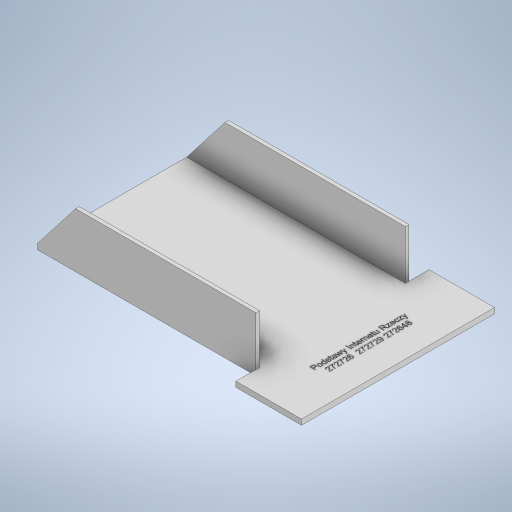
# Autodesk Inventor part: Część1
Saved by Autodesk Inventor 2024 (Build 280153020, 153B)
## iProperties
Created: 2025-01-23
Part Number: Część1
Material: Ogólny
Document SubType Name: Modeling
Designer: jakub
Density: 1 g/cm^3
Appearance: Domyślna
Author: jakub
Autodesk Inventor part; units mm, degrees
(part 1 of 2)
ref_plane "YZ Plane" through (0, 0, 0) normal (1, 0, 0) x (0, 1, 0)
ref_plane "XZ Plane" through (0, 0, 0) normal (0, 1, 0) x (-1, 0, 0)
ref_plane "XY Plane" through (0, 0, 0) normal (0, 0, 1) x (1, 0, 0)
sketch "Szkic1" plane through (0, 0, 0) normal (0, 1, 0) x (-1, 0, 0)
  line L0 (-24, 40) -> (60, 40)
  line L1 (60, -40) -> (-24, -40)
  line L2 (-60, -40) -> (-60, 40)
  line L3 (-60, 40) -> (60, -40) construction
  line L4 (60, 40) -> (-60, -40) construction
  line L5 (-24, -40) -> (-24, -53)
  line L6 (-24, -53) -> (-60, -53)
  line L7 (-60, -53) -> (-60, -40)
  line L8 (-24, 40) -> (-24, 53)
  line L9 (-24, 53) -> (-60, 53)
  line L10 (-60, 53) -> (-60, 40)
  line L11 (60, -40) -> (96, -40)
  line L12 (96, -40) -> (96, 40)
  line L13 (96, 40) -> (60, 40)
  point P0 (0, 0)
  dimension "d0" = 120
  dimension "d1" = 80
  dimension "d6" = 106
  dimension "d7" = 84
  dimension "d8" = 84
  dimension "d9" = 13
  dimension "d10" = 13
  dimension "d11" = 40
  dimension "d12" = 53
  dimension "d16" = 36
  dimension "d17" = 80
  dimension "d18" = 156
  constraints: 28 end point, 4 parallel, 2 horizontal, 2 midpoint, 1 perpendicular
  measures "d0" distance of L1.start L2.start
  measures "d1" distance of L0.end L1.start
  measures "d6" distance between parallel lines of L6 L9
  measures "d7" distance of L0.start L0.end
  measures "d8" distance of L1.start L1.end
  measures "d9" distance of L0.start L8.end
  measures "d10" distance of L1.end L5.end
  measures "d11" distance from line of point (0, 0) L1
  measures "d12" distance from line of point (0, 0) L9
  measures "d16" distance of L13.end L12.end
  measures "d17" distance of L11.end L12.end
  measures "d18" distance between parallel lines of L2 L12
extrude "Wyciągnięcie proste1" add sketch "Szkic1" along normal blind 3
sketch "Szkic2" plane through (0, 0, 0) normal (0, -1, 0) x (1, 0, 0)
  line L0 (24, -40) -> (-96, -40)
  line L1 (-96, -40) -> (-96, -42)
  line L2 (-96, -42) -> (24, -42)
  line L3 (24, -42) -> (24, -40)
  line L4 (24, 40) -> (-96, 40)
  line L5 (-96, 40) -> (-96, 42)
  line L6 (-96, 42) -> (24, 42)
  line L7 (24, 42) -> (24, 40)
  point P0 (0, 0)
  dimension "d19" = 2
  dimension "d20" = 120
  dimension "d21" = 2
  constraints: 16 end point, 4 parallel, 2 horizontal, 2 perpendicular, 1 point on line
  measures "d19" distance of L1.end L0.end
  measures "d20" distance of L5.end L6.end
  measures "d21" distance of L4.end L5.end
extrude "Wyciągnięcie proste2" add sketch "Szkic2" against normal blind 30
sketch "Szkic7" plane through (-96, 3, -40) normal (0, 0, 1) x (1, 0, 0)
  line L0 (0, 27) -> (120, 27) projected
  line L1 (0, 0) -> (21, 27)
  line L2 (0, 27) -> (21, 27)
  line L3 (0, 0) -> (0, 27)
  point P0 (96, -3)
  constraints: 6 end point, 1 perpendicular, 1 point on line
extrude "Wyciągnięcie proste4" cut sketch "Szkic7" along normal mid plane 200
sketch "Szkic8" plane through (0, 3, 0) normal (0, 1, 0) x (1, 0, 0)
  line L0 (37.3604, -27.9644) -> (37.3604, 27.055) construction
  line L1 (37.3604, 27.055) -> (143.5342, 27.055) construction
  line L2 (143.5342, 27.055) -> (143.5342, -27.9644) construction
  line L3 (143.5342, -27.9644) -> (37.3604, -27.9644) construction
  line L4 (40.4104, -25.9403) -> (37.3604, -25.9403)
  line L5 (37.3604, -25.9403) -> (37.3604, -24.7896)
  spline S0 degree 2 poles (37.3604, -24.7896) (37.3604, -24.4851) (37.3907, -24.3247) knots 0 0 0 1 1 1
  spline S1 degree 2 poles (37.3907, -24.3247) (37.4278, -24.0992) (37.6371, -23.797) (38.016, -23.611) (38.2438, -23.611) knots 0 0 0 1 2 3 3 3
  spline S2 degree 2 poles (38.2438, -23.611) (38.632, -23.611) (39.1714, -24.1062) (39.1714, -24.7524) knots 0 0 0 1 2 2 2
  line L6 (39.1714, -24.7524) -> (39.1714, -25.5358)
  line L7 (39.1714, -25.5358) -> (40.4104, -25.5358)
  line L8 (40.4104, -25.5358) -> (40.4104, -25.9403)
  line L9 (38.811, -25.5358) -> (38.811, -24.7478)
  spline S3 degree 2 poles (38.811, -24.7478) (38.811, -24.3549) (38.5205, -24.0271) (38.2554, -24.0271) knots 0 0 0 1 2 2 2
  spline S4 degree 2 poles (38.2554, -24.0271) (38.0648, -24.0271) (37.7905, -24.2201) (37.7487, -24.3781) knots 0 0 0 1 2 2 2
  spline S5 degree 2 poles (37.7487, -24.3781) (37.7208, -24.4804) (37.7208, -24.7547) knots 0 0 0 1 1 1
  line L10 (37.7208, -24.7547) -> (37.7208, -25.5358)
  line L11 (37.7208, -25.5358) -> (38.811, -25.5358)
  spline S6 degree 2 poles (39.3039, -23.2832) (38.6925, -23.2832) (38.3972, -22.9415) knots 0 0 0 1 1 1
  spline S7 degree 2 poles (38.3972, -22.9415) (38.1508, -22.6579) (38.1508, -22.2487) knots 0 0 0 1 1 1
  spline S8 degree 2 poles (38.1508, -22.2487) (38.1508, -21.7931) (38.7483, -21.2142) (39.2737, -21.2142) knots 0 0 0 1 2 2 2
  spline S9 degree 2 poles (39.2737, -21.2142) (39.6991, -21.2142) (40.1896, -21.47) (40.4592, -21.9581) (40.4592, -22.2487) knots 0 0 0 1 2 3 3 3
  spline S10 degree 2 poles (40.4592, -22.2487) (40.4592, -22.7113) (39.8641, -23.2832) (39.3039, -23.2832) knots 0 0 0 1 2 2 2
  spline S11 degree 2 poles (39.3062, -22.8973) (39.7293, -22.8973) (40.1524, -22.5277) (40.1524, -22.2487) knots 0 0 0 1 2 2 2
  spline S12 degree 2 poles (40.1524, -22.2487) (40.1524, -21.9698) (39.727, -21.6001) (39.2923, -21.6001) knots 0 0 0 1 2 2 2
  spline S13 degree 2 poles (39.2923, -21.6001) (38.8831, -21.6001) (38.46, -21.9721) (38.46, -22.2487) knots 0 0 0 1 2 2 2
  spline S14 degree 2 poles (38.46, -22.2487) (38.46, -22.5277) (38.8808, -22.8973) (39.3062, -22.8973) knots 0 0 0 1 2 2 2
  line L12 (40.4104, -19.3405) -> (40.1315, -19.3405)
  spline S15 degree 2 poles (40.1315, -19.3405) (40.4592, -19.5498) (40.4592, -19.9589) knots 0 0 0 1 1 1
  spline S16 degree 2 poles (40.4592, -19.9589) (40.4592, -20.2239) (40.1687, -20.6656) (39.6456, -20.9097) (39.3062, -20.9097) knots 0 0 0 1 2 3 3 3
  spline S17 degree 2 poles (39.3062, -20.9097) (38.9761, -20.9097) (38.4368, -20.6889) (38.1508, -20.2495) (38.1508, -19.9775) knots 0 0 0 1 2 3 3 3
  spline S18 degree 2 poles (38.1508, -19.9775) (38.1508, -19.7776) (38.3182, -19.4661) (38.453, -19.3684) knots 0 0 0 1 2 2 2
  line L13 (38.453, -19.3684) -> (37.3604, -19.3684)
  line L14 (37.3604, -19.3684) -> (37.3604, -18.9941)
  line L15 (37.3604, -18.9941) -> (40.4104, -18.9941)
  line L16 (40.4104, -18.9941) -> (40.4104, -19.3405)
  spline S19 degree 2 poles (39.3062, -20.5238) (39.7316, -20.5238) (40.1524, -20.1658) (40.1524, -19.9217) knots 0 0 0 1 2 2 2
  spline S20 degree 2 poles (40.1524, -19.9217) (40.1524, -19.6776) (39.7502, -19.3336) (39.3387, -19.3336) knots 0 0 0 1 2 2 2
  spline S21 degree 2 poles (39.3387, -19.3336) (38.8854, -19.3336) (38.46, -19.6823) (38.46, -19.938) knots 0 0 0 1 2 2 2
  spline S22 degree 2 poles (38.46, -19.938) (38.46, -20.189) (38.8692, -20.5238) (39.3062, -20.5238) knots 0 0 0 1 2 2 2
  line L17 (39.7502, -18.5571) -> (39.6921, -18.1875)
  spline S23 degree 2 poles (39.6921, -18.1875) (39.9153, -18.1573) (40.1524, -17.8713) (40.1524, -17.6133) knots 0 0 0 1 2 2 2
  spline S24 degree 2 poles (40.1524, -17.6133) (40.1524, -17.3552) (39.9408, -17.1042) (39.799, -17.1042) knots 0 0 0 1 2 2 2
  spline S25 degree 2 poles (39.799, -17.1042) (39.6735, -17.1042) (39.5991, -17.2158) knots 0 0 0 1 1 1
  spline S26 degree 2 poles (39.5991, -17.2158) (39.5503, -17.2925) (39.4736, -17.5993) knots 0 0 0 1 1 1
  spline S27 degree 2 poles (39.4736, -17.5993) (39.369, -18.0108) (39.2179, -18.3293) (38.9482, -18.4943) (38.7878, -18.4943) knots 0 0 0 1 2 3 3 3
  spline S28 degree 2 poles (38.7878, -18.4943) (38.639, -18.4943) (38.3879, -18.3595) (38.3043, -18.2433) knots 0 0 0 1 2 2 2
  spline S29 degree 2 poles (38.3043, -18.2433) (38.2392, -18.1549) (38.1508, -17.8527) (38.1508, -17.6784) knots 0 0 0 1 2 2 2
  spline S30 degree 2 poles (38.1508, -17.6784) (38.1508, -17.418) (38.3019, -17.0251) (38.5576, -16.8368) (38.7715, -16.802) knots 0 0 0 1 2 3 3 3
  line L18 (38.7715, -16.802) -> (38.8203, -17.1693)
  spline S31 degree 2 poles (38.8203, -17.1693) (38.6483, -17.1948) (38.4577, -17.4343) (38.4577, -17.6528) knots 0 0 0 1 2 2 2
  spline S32 degree 2 poles (38.4577, -17.6528) (38.4577, -17.9108) (38.6297, -18.1317) (38.7436, -18.1317) knots 0 0 0 1 2 2 2
  spline S33 degree 2 poles (38.7436, -18.1317) (38.8157, -18.1317) (38.8738, -18.0852) knots 0 0 0 1 1 1
  spline S34 degree 2 poles (38.8738, -18.0852) (38.9342, -18.041) (38.9738, -17.9411) knots 0 0 0 1 1 1
  spline S35 degree 2 poles (38.9738, -17.9411) (38.9947, -17.8853) (39.0714, -17.611) knots 0 0 0 1 1 1
  spline S36 degree 2 poles (39.0714, -17.611) (39.176, -17.2134) (39.3109, -16.8973) (39.5689, -16.7183) (39.7618, -16.7183) knots 0 0 0 1 2 3 3 3
  spline S37 degree 2 poles (39.7618, -16.7183) (39.9478, -16.7183) (40.2779, -16.9368) (40.4592, -17.3506) (40.4592, -17.611) knots 0 0 0 1 2 3 3 3
  spline S38 degree 2 poles (40.4592, -17.611) (40.4592, -18.041) (40.1012, -18.4943) (39.7502, -18.5571) knots 0 0 0 1 2 2 2
  line L19 (40.0757, -15.4583) -> (40.4081, -15.4048)
  spline S39 degree 2 poles (40.4081, -15.4048) (40.4407, -15.5629) (40.4407, -15.6884) knots 0 0 0 1 1 1
  spline S40 degree 2 poles (40.4407, -15.6884) (40.4407, -15.8907) (40.3105, -16.1162) (40.1012, -16.2068) (39.7642, -16.2068) knots 0 0 0 1 2 3 3 3
  line L20 (39.7642, -16.2068) -> (38.4902, -16.2068)
  line L21 (38.4902, -16.2068) -> (38.4902, -16.4835)
  line L22 (38.4902, -16.4835) -> (38.1996, -16.4835)
  line L23 (38.1996, -16.4835) -> (38.1996, -16.2068)
  line L24 (38.1996, -16.2068) -> (37.6533, -16.2068)
  line L25 (37.6533, -16.2068) -> (37.4278, -15.8326)
  line L26 (37.4278, -15.8326) -> (38.1996, -15.8326)
  line L27 (38.1996, -15.8326) -> (38.1996, -15.4583)
  line L28 (38.1996, -15.4583) -> (38.4902, -15.4583)
  line L29 (38.4902, -15.4583) -> (38.4902, -15.8326)
  line L30 (38.4902, -15.8326) -> (39.7851, -15.8326)
  spline S41 degree 2 poles (39.7851, -15.8326) (39.9455, -15.8326) (40.0385, -15.793) (40.0919, -15.7047) (40.0919, -15.621) knots 0 0 0 1 2 3 3 3
  spline S42 degree 2 poles (40.0919, -15.621) (40.0919, -15.5606) (40.0757, -15.4583) knots 0 0 0 1 1 1
  spline S43 degree 2 poles (40.1384, -13.6497) (40.3151, -13.8589) (40.4592, -14.2425) (40.4592, -14.4633) knots 0 0 0 1 2 2 2
  spline S44 degree 2 poles (40.4592, -14.4633) (40.4592, -14.8283) (40.1036, -15.2188) (39.8269, -15.2188) knots 0 0 0 1 2 2 2
  spline S45 degree 2 poles (39.8269, -15.2188) (39.6642, -15.2188) (39.3969, -15.0701) (39.2341, -14.8329) (39.1946, -14.6818) knots 0 0 0 1 2 3 3 3
  spline S46 degree 2 poles (39.1946, -14.6818) (39.1644, -14.5726) (39.1365, -14.3494) knots 0 0 0 1 1 1
  spline S47 degree 2 poles (39.1365, -14.3494) (39.083, -13.8961) (39.0086, -13.6822) knots 0 0 0 1 1 1
  spline S48 degree 2 poles (39.0086, -13.6822) (38.9319, -13.6799) (38.911, -13.6799) knots 0 0 0 1 1 1
  spline S49 degree 2 poles (38.911, -13.6799) (38.6809, -13.6799) (38.5879, -13.7868) knots 0 0 0 1 1 1
  spline S50 degree 2 poles (38.5879, -13.7868) (38.46, -13.9286) (38.46, -14.2123) knots 0 0 0 1 1 1
  spline S51 degree 2 poles (38.46, -14.2123) (38.46, -14.4749) (38.646, -14.726) (38.8808, -14.7865) knots 0 0 0 1 2 2 2
  line L31 (38.8808, -14.7865) -> (38.832, -15.1538)
  spline S52 degree 2 poles (38.832, -15.1538) (38.5972, -15.1049) (38.3066, -14.8748) (38.1508, -14.4424) (38.1508, -14.1588) knots 0 0 0 1 2 3 3 3
  spline S53 degree 2 poles (38.1508, -14.1588) (38.1508, -13.8752) (38.2833, -13.5218) (38.4856, -13.3544) (38.639, -13.3219) knots 0 0 0 1 2 3 3 3
  spline S54 degree 2 poles (38.639, -13.3219) (38.7367, -13.3033) (38.9854, -13.3033) knots 0 0 0 1 1 1
  line L32 (38.9854, -13.3033) -> (39.4852, -13.3033)
  spline S55 degree 2 poles (39.4852, -13.3033) (40.0059, -13.3033) (40.2826, -13.2545) (40.4104, -13.1847) knots 0 0 0 1 2 2 2
  line L33 (40.4104, -13.1847) -> (40.4104, -13.5753)
  spline S56 degree 2 poles (40.4104, -13.5753) (40.2942, -13.6334) (40.1384, -13.6497) knots 0 0 0 1 1 1
  spline S57 degree 2 poles (39.3016, -13.6799) (39.3852, -13.8845) (39.4434, -14.2913) knots 0 0 0 1 1 1
  spline S58 degree 2 poles (39.4434, -14.2913) (39.4759, -14.5238) (39.5596, -14.7144) (39.72, -14.819) (39.8176, -14.819) knots 0 0 0 1 2 3 3 3
  spline S59 degree 2 poles (39.8176, -14.819) (39.9664, -14.819) (40.1663, -14.5935) (40.1663, -14.375) knots 0 0 0 1 2 2 2
  spline S60 degree 2 poles (40.1663, -14.375) (40.1663, -14.1588) (39.978, -13.8217) (39.813, -13.7427) knots 0 0 0 1 2 2 2
  spline S61 degree 2 poles (39.813, -13.7427) (39.6851, -13.6822) (39.4387, -13.6822) knots 0 0 0 1 1 1
  line L34 (39.4387, -13.6822) -> (39.3016, -13.6799)
  line L35 (40.4104, -12.3199) -> (38.1996, -12.9918)
  line L36 (38.1996, -12.9918) -> (38.1996, -12.6059)
  line L37 (38.1996, -12.6059) -> (39.4759, -12.2525)
  line L38 (39.4759, -12.2525) -> (39.9501, -12.1247)
  spline S62 degree 2 poles (39.9501, -12.1247) (39.9153, -12.1154) (39.4945, -12.0084) knots 0 0 0 1 1 1
  line L39 (39.4945, -12.0084) -> (38.1996, -11.6574)
  line L40 (38.1996, -11.6574) -> (38.1996, -11.2715)
  line L41 (38.1996, -11.2715) -> (39.4829, -10.9414)
  line L42 (39.4829, -10.9414) -> (39.9036, -10.8321)
  line L43 (39.9036, -10.8321) -> (39.4759, -10.7066)
  line L44 (39.4759, -10.7066) -> (38.1996, -10.3254)
  line L45 (38.1996, -10.3254) -> (38.1996, -9.9604)
  line L46 (38.1996, -9.9604) -> (40.4104, -10.6555)
  line L47 (40.4104, -10.6555) -> (40.4104, -11.0414)
  line L48 (40.4104, -11.0414) -> (39.0877, -11.3924)
  line L49 (39.0877, -11.3924) -> (38.7088, -11.4784)
  line L50 (38.7088, -11.4784) -> (40.4104, -11.9294)
  line L51 (40.4104, -11.9294) -> (40.4104, -12.3199)
  line L52 (41.2589, -9.6605) -> (40.9079, -9.7023)
  spline S63 degree 2 poles (40.9079, -9.7023) (40.9405, -9.5791) (40.9405, -9.4885) knots 0 0 0 1 1 1
  spline S64 degree 2 poles (40.9405, -9.4885) (40.9405, -9.3629) (40.8568, -9.2142) (40.7824, -9.1653) knots 0 0 0 1 2 2 2
  spline S65 degree 2 poles (40.7824, -9.1653) (40.7266, -9.1305) (40.5034, -9.0514) knots 0 0 0 1 1 1
  spline S66 degree 2 poles (40.5034, -9.0514) (40.4732, -9.0421) (40.4128, -9.0189) knots 0 0 0 1 1 1
  line L53 (40.4128, -9.0189) -> (38.1996, -9.8581)
  line L54 (38.1996, -9.8581) -> (38.1996, -9.4536)
  line L55 (38.1996, -9.4536) -> (39.4759, -8.9956)
  spline S67 degree 2 poles (39.4759, -8.9956) (39.7177, -8.905) (39.985, -8.8352) knots 0 0 0 1 1 1
  spline S68 degree 2 poles (39.985, -8.8352) (39.7339, -8.7701) (39.4875, -8.6795) knots 0 0 0 1 1 1
  line L56 (39.4875, -8.6795) -> (38.1996, -8.2076)
  line L57 (38.1996, -8.2076) -> (38.1996, -7.8333)
  line L58 (38.1996, -7.8333) -> (40.45, -8.6725)
  spline S69 degree 2 poles (40.45, -8.6725) (40.8126, -8.8073) (40.9498, -8.8817) knots 0 0 0 1 1 1
  spline S70 degree 2 poles (40.9498, -8.8817) (41.1334, -8.9817) (41.3054, -9.2397) (41.3054, -9.4187) knots 0 0 0 1 2 2 2
  spline S71 degree 2 poles (41.3054, -9.4187) (41.3054, -9.528) (41.2589, -9.6605) knots 0 0 0 1 1 1
  line L59 (40.4104, -6.213) -> (37.3604, -6.213)
  line L60 (37.3604, -6.213) -> (37.3604, -5.8085)
  line L61 (37.3604, -5.8085) -> (40.4104, -5.8085)
  line L62 (40.4104, -5.8085) -> (40.4104, -6.213)
  line L63 (40.4104, -5.1459) -> (38.1996, -5.1459)
  line L64 (38.1996, -5.1459) -> (38.1996, -4.8089)
  line L65 (38.1996, -4.8089) -> (38.5135, -4.8089)
  spline S72 degree 2 poles (38.5135, -4.8089) (38.1508, -4.5648) (38.1508, -4.1068) knots 0 0 0 1 1 1
  spline S73 degree 2 poles (38.1508, -4.1068) (38.1508, -3.9069) (38.295, -3.5721) (38.5274, -3.4047) (38.6878, -3.3722) knots 0 0 0 1 2 3 3 3
  spline S74 degree 2 poles (38.6878, -3.3722) (38.7924, -3.3513) (39.0528, -3.3513) knots 0 0 0 1 1 1
  line L66 (39.0528, -3.3513) -> (40.4104, -3.3513)
  line L67 (40.4104, -3.3513) -> (40.4104, -3.7256)
  line L68 (40.4104, -3.7256) -> (39.0668, -3.7256)
  spline S75 degree 2 poles (39.0668, -3.7256) (38.8389, -3.7256) (38.6111, -3.8139) (38.4763, -4.0347) (38.4763, -4.1858) knots 0 0 0 1 2 3 3 3
  spline S76 degree 2 poles (38.4763, -4.1858) (38.4763, -4.4253) (38.7808, -4.7717) (39.2039, -4.7717) knots 0 0 0 1 2 2 2
  line L69 (39.2039, -4.7717) -> (40.4104, -4.7717)
  line L70 (40.4104, -4.7717) -> (40.4104, -5.1459)
  line L71 (40.0757, -1.9611) -> (40.4081, -1.9076)
  spline S77 degree 2 poles (40.4081, -1.9076) (40.4407, -2.0657) (40.4407, -2.1913) knots 0 0 0 1 1 1
  spline S78 degree 2 poles (40.4407, -2.1913) (40.4407, -2.3935) (40.3105, -2.619) (40.1012, -2.7097) (39.7642, -2.7097) knots 0 0 0 1 2 3 3 3
  line L72 (39.7642, -2.7097) -> (38.4902, -2.7097)
  line L73 (38.4902, -2.7097) -> (38.4902, -2.9863)
  line L74 (38.4902, -2.9863) -> (38.1996, -2.9863)
  line L75 (38.1996, -2.9863) -> (38.1996, -2.7097)
  line L76 (38.1996, -2.7097) -> (37.6533, -2.7097)
  line L77 (37.6533, -2.7097) -> (37.4278, -2.3354)
  line L78 (37.4278, -2.3354) -> (38.1996, -2.3354)
  line L79 (38.1996, -2.3354) -> (38.1996, -1.9611)
  line L80 (38.1996, -1.9611) -> (38.4902, -1.9611)
  line L81 (38.4902, -1.9611) -> (38.4902, -2.3354)
  line L82 (38.4902, -2.3354) -> (39.7851, -2.3354)
  spline S79 degree 2 poles (39.7851, -2.3354) (39.9455, -2.3354) (40.0385, -2.2959) (40.0919, -2.2075) (40.0919, -2.1238) knots 0 0 0 1 2 3 3 3
  spline S80 degree 2 poles (40.0919, -2.1238) (40.0919, -2.0634) (40.0757, -1.9611) knots 0 0 0 1 1 1
  line L83 (39.6967, -0.0828) -> (39.7456, 0.3055)
  spline S81 degree 2 poles (39.7456, 0.3055) (40.085, 0.2125) (40.4592, -0.2827) (40.4592, -0.6663) knots 0 0 0 1 2 2 2
  spline S82 degree 2 poles (40.4592, -0.6663) (40.4592, -1.1521) (39.8618, -1.7193) (39.3248, -1.7193) knots 0 0 0 1 2 2 2
  spline S83 degree 2 poles (39.3248, -1.7193) (38.7669, -1.7193) (38.1508, -1.1451) (38.1508, -0.6872) knots 0 0 0 1 2 2 2
  spline S84 degree 2 poles (38.1508, -0.6872) (38.1508, -0.2455) (38.7552, 0.3171) (39.3016, 0.3171) knots 0 0 0 1 2 2 2
  spline S85 degree 2 poles (39.3016, 0.3171) (39.3341, 0.3171) (39.4015, 0.3148) knots 0 0 0 1 1 1
  line L84 (39.4015, 0.3148) -> (39.4015, -1.3334)
  spline S86 degree 2 poles (39.4015, -1.3334) (39.7665, -1.3125) (40.1524, -0.9429) (40.1524, -0.6663) knots 0 0 0 1 2 2 2
  spline S87 degree 2 poles (40.1524, -0.6663) (40.1524, -0.4594) (39.9339, -0.1688) (39.6967, -0.0828) knots 0 0 0 1 2 2 2
  line L85 (39.0947, -1.3125) -> (39.0947, -0.0781)
  spline S88 degree 2 poles (39.0947, -0.0781) (38.8157, -0.1037) (38.6739, -0.2199) knots 0 0 0 1 1 1
  spline S89 degree 2 poles (38.6739, -0.2199) (38.4577, -0.3989) (38.4577, -0.6849) knots 0 0 0 1 1 1
  spline S90 degree 2 poles (38.4577, -0.6849) (38.4577, -0.9429) (38.8041, -1.2939) (39.0947, -1.3125) knots 0 0 0 1 2 2 2
  line L86 (40.4104, 0.7704) -> (38.1996, 0.7704)
  line L87 (38.1996, 0.7704) -> (38.1996, 1.1075)
  line L88 (38.1996, 1.1075) -> (38.5344, 1.1075)
  spline S91 degree 2 poles (38.5344, 1.1075) (38.2996, 1.2353) (38.1508, 1.4539) (38.1508, 1.5864) knots 0 0 0 1 2 2 2
  spline S92 degree 2 poles (38.1508, 1.5864) (38.1508, 1.7747) (38.2694, 1.97) knots 0 0 0 1 1 1
  line L89 (38.2694, 1.97) -> (38.6181, 1.8398)
  spline S93 degree 2 poles (38.6181, 1.8398) (38.5367, 1.7026) (38.5367, 1.5655) knots 0 0 0 1 1 1
  spline S94 degree 2 poles (38.5367, 1.5655) (38.5367, 1.4422) (38.6855, 1.2493) (38.8157, 1.2075) knots 0 0 0 1 2 2 2
  spline S95 degree 2 poles (38.8157, 1.2075) (39.0156, 1.1447) (39.2527, 1.1447) knots 0 0 0 1 1 1
  line L90 (39.2527, 1.1447) -> (40.4104, 1.1447)
  line L91 (40.4104, 1.1447) -> (40.4104, 0.7704)
  line L92 (40.4104, 2.1931) -> (38.1996, 2.1931)
  line L93 (38.1996, 2.1931) -> (38.1996, 2.5302)
  line L94 (38.1996, 2.5302) -> (38.5135, 2.5302)
  spline S96 degree 2 poles (38.5135, 2.5302) (38.1508, 2.7743) (38.1508, 3.2323) knots 0 0 0 1 1 1
  spline S97 degree 2 poles (38.1508, 3.2323) (38.1508, 3.4322) (38.295, 3.7669) (38.5274, 3.9343) (38.6878, 3.9669) knots 0 0 0 1 2 3 3 3
  spline S98 degree 2 poles (38.6878, 3.9669) (38.7924, 3.9878) (39.0528, 3.9878) knots 0 0 0 1 1 1
  line L95 (39.0528, 3.9878) -> (40.4104, 3.9878)
  line L96 (40.4104, 3.9878) -> (40.4104, 3.6135)
  line L97 (40.4104, 3.6135) -> (39.0668, 3.6135)
  spline S99 degree 2 poles (39.0668, 3.6135) (38.8389, 3.6135) (38.6111, 3.5252) (38.4763, 3.3043) (38.4763, 3.1532) knots 0 0 0 1 2 3 3 3
  spline S100 degree 2 poles (38.4763, 3.1532) (38.4763, 2.9138) (38.7808, 2.5674) (39.2039, 2.5674) knots 0 0 0 1 2 2 2
  line L98 (39.2039, 2.5674) -> (40.4104, 2.5674)
  line L99 (40.4104, 2.5674) -> (40.4104, 2.1931)
  line L100 (39.6967, 6.073) -> (39.7456, 6.4613)
  spline S101 degree 2 poles (39.7456, 6.4613) (40.085, 6.3683) (40.4592, 5.8731) (40.4592, 5.4895) knots 0 0 0 1 2 2 2
  spline S102 degree 2 poles (40.4592, 5.4895) (40.4592, 5.0037) (39.8618, 4.4365) (39.3248, 4.4365) knots 0 0 0 1 2 2 2
  spline S103 degree 2 poles (39.3248, 4.4365) (38.7669, 4.4365) (38.1508, 5.0107) (38.1508, 5.4686) knots 0 0 0 1 2 2 2
  spline S104 degree 2 poles (38.1508, 5.4686) (38.1508, 5.9103) (38.7552, 6.4729) (39.3016, 6.4729) knots 0 0 0 1 2 2 2
  spline S105 degree 2 poles (39.3016, 6.4729) (39.3341, 6.4729) (39.4015, 6.4706) knots 0 0 0 1 1 1
  line L101 (39.4015, 6.4706) -> (39.4015, 4.8224)
  spline S106 degree 2 poles (39.4015, 4.8224) (39.7665, 4.8433) (40.1524, 5.2129) (40.1524, 5.4895) knots 0 0 0 1 2 2 2
  spline S107 degree 2 poles (40.1524, 5.4895) (40.1524, 5.6964) (39.9339, 5.987) (39.6967, 6.073) knots 0 0 0 1 2 2 2
  line L102 (39.0947, 4.8433) -> (39.0947, 6.0777)
  spline S108 degree 2 poles (39.0947, 6.0777) (38.8157, 6.0521) (38.6739, 5.9359) knots 0 0 0 1 1 1
  spline S109 degree 2 poles (38.6739, 5.9359) (38.4577, 5.7569) (38.4577, 5.4709) knots 0 0 0 1 1 1
  spline S110 degree 2 poles (38.4577, 5.4709) (38.4577, 5.2129) (38.8041, 4.8619) (39.0947, 4.8433) knots 0 0 0 1 2 2 2
  line L103 (40.0757, 7.7468) -> (40.4081, 7.8003)
  spline S111 degree 2 poles (40.4081, 7.8003) (40.4407, 7.6422) (40.4407, 7.5167) knots 0 0 0 1 1 1
  spline S112 degree 2 poles (40.4407, 7.5167) (40.4407, 7.3144) (40.3105, 7.0889) (40.1012, 6.9983) (39.7642, 6.9983) knots 0 0 0 1 2 3 3 3
  line L104 (39.7642, 6.9983) -> (38.4902, 6.9983)
  line L105 (38.4902, 6.9983) -> (38.4902, 6.7216)
  line L106 (38.4902, 6.7216) -> (38.1996, 6.7216)
  line L107 (38.1996, 6.7216) -> (38.1996, 6.9983)
  line L108 (38.1996, 6.9983) -> (37.6533, 6.9983)
  line L109 (37.6533, 6.9983) -> (37.4278, 7.3725)
  line L110 (37.4278, 7.3725) -> (38.1996, 7.3725)
  line L111 (38.1996, 7.3725) -> (38.1996, 7.7468)
  line L112 (38.1996, 7.7468) -> (38.4902, 7.7468)
  line L113 (38.4902, 7.7468) -> (38.4902, 7.3725)
  line L114 (38.4902, 7.3725) -> (39.7851, 7.3725)
  spline S113 degree 2 poles (39.7851, 7.3725) (39.9455, 7.3725) (40.0385, 7.4121) (40.0919, 7.5004) (40.0919, 7.5841) knots 0 0 0 1 2 3 3 3
  spline S114 degree 2 poles (40.0919, 7.5841) (40.0919, 7.6445) (40.0757, 7.7468) knots 0 0 0 1 1 1
  line L115 (40.4104, 9.5601) -> (40.085, 9.5601)
  spline S115 degree 2 poles (40.085, 9.5601) (40.4592, 9.302) (40.4592, 8.8603) knots 0 0 0 1 1 1
  spline S116 degree 2 poles (40.4592, 8.8603) (40.4592, 8.6651) (40.3105, 8.3257) (40.0826, 8.1606) (39.9176, 8.1281) knots 0 0 0 1 2 3 3 3
  spline S117 degree 2 poles (39.9176, 8.1281) (39.8083, 8.1048) (39.5689, 8.1048) knots 0 0 0 1 1 1
  line L116 (39.5689, 8.1048) -> (38.1996, 8.1048)
  line L117 (38.1996, 8.1048) -> (38.1996, 8.4791)
  line L118 (38.1996, 8.4791) -> (39.4248, 8.4791)
  spline S118 degree 2 poles (39.4248, 8.4791) (39.7177, 8.4791) (39.82, 8.5023) knots 0 0 0 1 1 1
  spline S119 degree 2 poles (39.82, 8.5023) (39.9687, 8.5372) (40.1361, 8.765) (40.1361, 8.9347) knots 0 0 0 1 2 2 2
  spline S120 degree 2 poles (40.1361, 8.9347) (40.1361, 9.1021) (39.9641, 9.3974) (39.6665, 9.5206) (39.3829, 9.5206) knots 0 0 0 1 2 3 3 3
  line L119 (39.3829, 9.5206) -> (38.1996, 9.5206)
  line L120 (38.1996, 9.5206) -> (38.1996, 9.8948)
  line L121 (38.1996, 9.8948) -> (40.4104, 9.8948)
  line L122 (40.4104, 9.8948) -> (40.4104, 9.5601)
  line L123 (40.4104, 11.7197) -> (37.3604, 11.7197)
  line L124 (37.3604, 11.7197) -> (37.3604, 13.0727)
  spline S121 degree 2 poles (37.3604, 13.0727) (37.3604, 13.4795) (37.5255, 13.9049) (37.9416, 14.1583) (38.1927, 14.1583) knots 0 0 0 1 2 3 3 3
  spline S122 degree 2 poles (38.1927, 14.1583) (38.5181, 14.1583) (38.9621, 13.7376) (39.0226, 13.3005) knots 0 0 0 1 2 2 2
  spline S123 degree 2 poles (39.0226, 13.3005) (39.0993, 13.4586) (39.1737, 13.5423) knots 0 0 0 1 1 1
  spline S124 degree 2 poles (39.1737, 13.5423) (39.3364, 13.719) (39.5805, 13.877) knots 0 0 0 1 1 1
  line L125 (39.5805, 13.877) -> (40.4104, 14.4047)
  line L126 (40.4104, 14.4047) -> (40.4104, 13.9003)
  line L127 (40.4104, 13.9003) -> (39.7758, 13.4958)
  spline S125 degree 2 poles (39.7758, 13.4958) (39.5015, 13.3191) (39.2109, 13.0913) (39.0923, 12.91) (39.0691, 12.817) knots 0 0 0 1 2 3 3 3
  spline S126 degree 2 poles (39.0691, 12.817) (39.0551, 12.7472) (39.0551, 12.5915) knots 0 0 0 1 1 1
  line L128 (39.0551, 12.5915) -> (39.0551, 12.1242)
  line L129 (39.0551, 12.1242) -> (40.4104, 12.1242)
  line L130 (40.4104, 12.1242) -> (40.4104, 11.7197)
  line L131 (38.7064, 12.1242) -> (38.7064, 12.9913)
  spline S127 degree 2 poles (38.7064, 12.9913) (38.7064, 13.268) (38.5925, 13.5795) (38.3391, 13.7422) (38.1927, 13.7422) knots 0 0 0 1 2 3 3 3
  spline S128 degree 2 poles (38.1927, 13.7422) (37.9765, 13.7422) (37.6975, 13.4284) (37.6975, 13.089) knots 0 0 0 1 2 2 2
  line L132 (37.6975, 13.089) -> (37.6975, 12.1242)
  line L133 (37.6975, 12.1242) -> (38.7064, 12.1242)
  line L134 (40.4104, 14.5466) -> (40.1059, 14.5466)
  line L135 (40.1059, 14.5466) -> (38.4926, 15.9507)
  spline S129 degree 2 poles (38.4926, 15.9507) (38.5042, 15.7112) (38.5042, 15.5276) knots 0 0 0 1 1 1
  line L136 (38.5042, 15.5276) -> (38.5042, 14.6302)
  line L137 (38.5042, 14.6302) -> (38.1996, 14.6302)
  line L138 (38.1996, 14.6302) -> (38.1996, 16.4342)
  line L139 (38.1996, 16.4342) -> (38.4484, 16.4342)
  line L140 (38.4484, 16.4342) -> (39.8502, 15.237)
  line L141 (39.8502, 15.237) -> (40.1059, 15.0092)
  spline S130 degree 2 poles (40.1059, 15.0092) (40.0873, 15.2602) (40.0873, 15.4811) knots 0 0 0 1 1 1
  line L142 (40.0873, 15.4811) -> (40.0873, 16.5016)
  line L143 (40.0873, 16.5016) -> (40.4104, 16.5016)
  line L144 (40.4104, 16.5016) -> (40.4104, 14.5466)
  line L145 (39.6967, 18.3869) -> (39.7456, 18.7752)
  spline S131 degree 2 poles (39.7456, 18.7752) (40.085, 18.6822) (40.4592, 18.187) (40.4592, 17.8035) knots 0 0 0 1 2 2 2
  spline S132 degree 2 poles (40.4592, 17.8035) (40.4592, 17.3176) (39.8618, 16.7504) (39.3248, 16.7504) knots 0 0 0 1 2 2 2
  spline S133 degree 2 poles (39.3248, 16.7504) (38.7669, 16.7504) (38.1508, 17.3246) (38.1508, 17.7825) knots 0 0 0 1 2 2 2
  spline S134 degree 2 poles (38.1508, 17.7825) (38.1508, 18.2242) (38.7552, 18.7868) (39.3016, 18.7868) knots 0 0 0 1 2 2 2
  spline S135 degree 2 poles (39.3016, 18.7868) (39.3341, 18.7868) (39.4015, 18.7845) knots 0 0 0 1 1 1
  line L146 (39.4015, 18.7845) -> (39.4015, 17.1363)
  spline S136 degree 2 poles (39.4015, 17.1363) (39.7665, 17.1572) (40.1524, 17.5268) (40.1524, 17.8035) knots 0 0 0 1 2 2 2
  spline S137 degree 2 poles (40.1524, 17.8035) (40.1524, 18.0103) (39.9339, 18.3009) (39.6967, 18.3869) knots 0 0 0 1 2 2 2
  line L147 (39.0947, 17.1572) -> (39.0947, 18.3916)
  spline S138 degree 2 poles (39.0947, 18.3916) (38.8157, 18.366) (38.6739, 18.2498) knots 0 0 0 1 1 1
  spline S139 degree 2 poles (38.6739, 18.2498) (38.4577, 18.0708) (38.4577, 17.7849) knots 0 0 0 1 1 1
  spline S140 degree 2 poles (38.4577, 17.7849) (38.4577, 17.5268) (38.8041, 17.1758) (39.0947, 17.1572) knots 0 0 0 1 2 2 2
  line L148 (39.6014, 20.6884) -> (39.6503, 21.0557)
  spline S141 degree 2 poles (39.6503, 21.0557) (40.0292, 20.9953) (40.4592, 20.4978) (40.4592, 20.1351) knots 0 0 0 1 2 2 2
  spline S142 degree 2 poles (40.4592, 20.1351) (40.4592, 19.6818) (39.8665, 19.1309) (39.3132, 19.1309) knots 0 0 0 1 2 2 2
  spline S143 degree 2 poles (39.3132, 19.1309) (38.9552, 19.1309) (38.4182, 19.368) (38.1508, 19.8538) (38.1508, 20.1374) knots 0 0 0 1 2 3 3 3
  spline S144 degree 2 poles (38.1508, 20.1374) (38.1508, 20.4978) (38.5158, 20.9557) (38.8506, 21.0208) knots 0 0 0 1 2 2 2
  line L149 (38.8506, 21.0208) -> (38.9064, 20.6559)
  spline S145 degree 2 poles (38.9064, 20.6559) (38.6832, 20.6047) (38.4577, 20.3397) (38.4577, 20.1537) knots 0 0 0 1 2 2 2
  spline S146 degree 2 poles (38.4577, 20.1537) (38.4577, 19.8701) (38.8645, 19.5168) (39.3039, 19.5168) knots 0 0 0 1 2 2 2
  spline S147 degree 2 poles (39.3039, 19.5168) (39.7479, 19.5168) (40.1524, 19.8585) (40.1524, 20.1328) knots 0 0 0 1 2 2 2
  spline S148 degree 2 poles (40.1524, 20.1328) (40.1524, 20.3536) (39.8827, 20.6489) (39.6014, 20.6884) knots 0 0 0 1 2 2 2
  line L150 (40.4104, 21.1789) -> (40.1059, 21.1789)
  line L151 (40.1059, 21.1789) -> (38.4926, 22.583)
  spline S149 degree 2 poles (38.4926, 22.583) (38.5042, 22.3436) (38.5042, 22.1599) knots 0 0 0 1 1 1
  line L152 (38.5042, 22.1599) -> (38.5042, 21.2626)
  line L153 (38.5042, 21.2626) -> (38.1996, 21.2626)
  line L154 (38.1996, 21.2626) -> (38.1996, 23.0666)
  line L155 (38.1996, 23.0666) -> (38.4484, 23.0666)
  line L156 (38.4484, 23.0666) -> (39.8502, 21.8693)
  line L157 (39.8502, 21.8693) -> (40.1059, 21.6415)
  spline S150 degree 2 poles (40.1059, 21.6415) (40.0873, 21.8926) (40.0873, 22.1134) knots 0 0 0 1 1 1
  line L158 (40.0873, 22.1134) -> (40.0873, 23.134)
  line L159 (40.0873, 23.134) -> (40.4104, 23.134)
  line L160 (40.4104, 23.134) -> (40.4104, 21.1789)
  line L161 (41.2589, 23.492) -> (40.9079, 23.4501)
  spline S151 degree 2 poles (40.9079, 23.4501) (40.9405, 23.5733) (40.9405, 23.664) knots 0 0 0 1 1 1
  spline S152 degree 2 poles (40.9405, 23.664) (40.9405, 23.7895) (40.8568, 23.9383) (40.7824, 23.9871) knots 0 0 0 1 2 2 2
  spline S153 degree 2 poles (40.7824, 23.9871) (40.7266, 24.022) (40.5034, 24.101) knots 0 0 0 1 1 1
  spline S154 degree 2 poles (40.5034, 24.101) (40.4732, 24.1103) (40.4128, 24.1336) knots 0 0 0 1 1 1
  line L162 (40.4128, 24.1336) -> (38.1996, 23.2944)
  line L163 (38.1996, 23.2944) -> (38.1996, 23.6989)
  line L164 (38.1996, 23.6989) -> (39.4759, 24.1568)
  spline S155 degree 2 poles (39.4759, 24.1568) (39.7177, 24.2475) (39.985, 24.3172) knots 0 0 0 1 1 1
  spline S156 degree 2 poles (39.985, 24.3172) (39.7339, 24.3823) (39.4875, 24.473) knots 0 0 0 1 1 1
  line L165 (39.4875, 24.473) -> (38.1996, 24.9449)
  line L166 (38.1996, 24.9449) -> (38.1996, 25.3192)
  line L167 (38.1996, 25.3192) -> (40.45, 24.48)
  spline S157 degree 2 poles (40.45, 24.48) (40.8126, 24.3451) (40.9498, 24.2708) knots 0 0 0 1 1 1
  spline S158 degree 2 poles (40.9498, 24.2708) (41.1334, 24.1708) (41.3054, 23.9127) (41.3054, 23.7337) knots 0 0 0 1 2 2 2
  spline S159 degree 2 poles (41.3054, 23.7337) (41.3054, 23.6245) (41.2589, 23.492) knots 0 0 0 1 1 1
  line L168 (44.8499, -20.8144) -> (45.2102, -20.8144)
  line L169 (45.2102, -20.8144) -> (45.2102, -22.8299)
  spline S160 degree 2 poles (45.2102, -22.8299) (45.0754, -22.8345) (44.9499, -22.7857) knots 0 0 0 1 1 1
  spline S161 degree 2 poles (44.9499, -22.7857) (44.743, -22.709) (44.3454, -22.3696) (44.0827, -22.0488) knots 0 0 0 1 2 2 2
  spline S162 degree 2 poles (44.0827, -22.0488) (43.6736, -21.5536) (43.1994, -21.2049) (42.9855, -21.2049) knots 0 0 0 1 2 2 2
  spline S163 degree 2 poles (42.9855, -21.2049) (42.7623, -21.2049) (42.4578, -21.5234) (42.4578, -21.7791) knots 0 0 0 1 2 2 2
  spline S164 degree 2 poles (42.4578, -21.7791) (42.4578, -22.0488) (42.7832, -22.3719) (43.0692, -22.3743) knots 0 0 0 1 2 2 2
  line L170 (43.0692, -22.3743) -> (43.0297, -22.7602)
  spline S165 degree 2 poles (43.0297, -22.7602) (42.5996, -22.7206) (42.1486, -22.2046) (42.1486, -21.7698) knots 0 0 0 1 2 2 2
  spline S166 degree 2 poles (42.1486, -21.7698) (42.1486, -21.3305) (42.6345, -20.819) (42.9948, -20.819) knots 0 0 0 1 2 2 2
  spline S167 degree 2 poles (42.9948, -20.819) (43.1784, -20.819) (43.5318, -20.9678) (43.9223, -21.3165) (44.2641, -21.7187) knots 0 0 0 1 2 3 3 3
  spline S168 degree 2 poles (44.2641, -21.7187) (44.5454, -22.0558) (44.7476, -22.2464) (44.8499, -22.3092) knots 0 0 0 1 2 2 2
  line L171 (44.8499, -22.3092) -> (44.8499, -20.8144)
  line L172 (42.5601, -20.3866) -> (42.1997, -20.3866)
  line L173 (42.1997, -20.3866) -> (42.1997, -18.413)
  line L174 (42.1997, -18.413) -> (42.4903, -18.413)
  spline S169 degree 2 poles (42.4903, -18.413) (42.8018, -18.7036) (43.8294, -19.2754) (44.371, -19.4312) knots 0 0 0 1 2 2 2
  spline S170 degree 2 poles (44.371, -19.4312) (44.7546, -19.5451) (45.2102, -19.5753) knots 0 0 0 1 1 1
  line L175 (45.2102, -19.5753) -> (45.2102, -19.9612)
  spline S171 degree 2 poles (45.2102, -19.9612) (44.8499, -19.9543) (43.8317, -19.6846) (42.8855, -19.1801) (42.5601, -18.8942) knots 0 0 0 1 2 3 3 3
  line L176 (42.5601, -18.8942) -> (42.5601, -20.3866)
  line L177 (44.8499, -16.0767) -> (45.2102, -16.0767)
  line L178 (45.2102, -16.0767) -> (45.2102, -18.0922)
  spline S172 degree 2 poles (45.2102, -18.0922) (45.0754, -18.0968) (44.9499, -18.048) knots 0 0 0 1 1 1
  spline S173 degree 2 poles (44.9499, -18.048) (44.743, -17.9713) (44.3454, -17.6319) (44.0827, -17.3111) knots 0 0 0 1 2 2 2
  spline S174 degree 2 poles (44.0827, -17.3111) (43.6736, -16.8159) (43.1994, -16.4672) (42.9855, -16.4672) knots 0 0 0 1 2 2 2
  spline S175 degree 2 poles (42.9855, -16.4672) (42.7623, -16.4672) (42.4578, -16.7857) (42.4578, -17.0414) knots 0 0 0 1 2 2 2
  spline S176 degree 2 poles (42.4578, -17.0414) (42.4578, -17.3111) (42.7832, -17.6342) (43.0692, -17.6365) knots 0 0 0 1 2 2 2
  line L179 (43.0692, -17.6365) -> (43.0297, -18.0224)
  spline S177 degree 2 poles (43.0297, -18.0224) (42.5996, -17.9829) (42.1486, -17.4668) (42.1486, -17.0321) knots 0 0 0 1 2 2 2
  spline S178 degree 2 poles (42.1486, -17.0321) (42.1486, -16.5927) (42.6345, -16.0813) (42.9948, -16.0813) knots 0 0 0 1 2 2 2
  spline S179 degree 2 poles (42.9948, -16.0813) (43.1784, -16.0813) (43.5318, -16.2301) (43.9223, -16.5788) (44.2641, -16.981) knots 0 0 0 1 2 3 3 3
  spline S180 degree 2 poles (44.2641, -16.981) (44.5454, -17.318) (44.7476, -17.5087) (44.8499, -17.5714) knots 0 0 0 1 2 2 2
  line L180 (44.8499, -17.5714) -> (44.8499, -16.0767)
  line L181 (42.5601, -15.6489) -> (42.1997, -15.6489)
  line L182 (42.1997, -15.6489) -> (42.1997, -13.6752)
  line L183 (42.1997, -13.6752) -> (42.4903, -13.6752)
  spline S181 degree 2 poles (42.4903, -13.6752) (42.8018, -13.9658) (43.8294, -14.5377) (44.371, -14.6935) knots 0 0 0 1 2 2 2
  spline S182 degree 2 poles (44.371, -14.6935) (44.7546, -14.8074) (45.2102, -14.8376) knots 0 0 0 1 1 1
  line L184 (45.2102, -14.8376) -> (45.2102, -15.2235)
  spline S183 degree 2 poles (45.2102, -15.2235) (44.8499, -15.2165) (43.8317, -14.9469) (42.8855, -14.4424) (42.5601, -14.1565) knots 0 0 0 1 2 3 3 3
  line L185 (42.5601, -14.1565) -> (42.5601, -15.6489)
  line L186 (44.8499, -11.3389) -> (45.2102, -11.3389)
  line L187 (45.2102, -11.3389) -> (45.2102, -13.3544)
  spline S184 degree 2 poles (45.2102, -13.3544) (45.0754, -13.3591) (44.9499, -13.3103) knots 0 0 0 1 1 1
  spline S185 degree 2 poles (44.9499, -13.3103) (44.743, -13.2336) (44.3454, -12.8942) (44.0827, -12.5733) knots 0 0 0 1 2 2 2
  spline S186 degree 2 poles (44.0827, -12.5733) (43.6736, -12.0782) (43.1994, -11.7295) (42.9855, -11.7295) knots 0 0 0 1 2 2 2
  spline S187 degree 2 poles (42.9855, -11.7295) (42.7623, -11.7295) (42.4578, -12.048) (42.4578, -12.3037) knots 0 0 0 1 2 2 2
  spline S188 degree 2 poles (42.4578, -12.3037) (42.4578, -12.5733) (42.7832, -12.8965) (43.0692, -12.8988) knots 0 0 0 1 2 2 2
  line L188 (43.0692, -12.8988) -> (43.0297, -13.2847)
  spline S189 degree 2 poles (43.0297, -13.2847) (42.5996, -13.2452) (42.1486, -12.7291) (42.1486, -12.2944) knots 0 0 0 1 2 2 2
  spline S190 degree 2 poles (42.1486, -12.2944) (42.1486, -11.855) (42.6345, -11.3436) (42.9948, -11.3436) knots 0 0 0 1 2 2 2
  spline S191 degree 2 poles (42.9948, -11.3436) (43.1784, -11.3436) (43.5318, -11.4924) (43.9223, -11.8411) (44.2641, -12.2432) knots 0 0 0 1 2 3 3 3
  spline S192 degree 2 poles (44.2641, -12.2432) (44.5454, -12.5803) (44.7476, -12.7709) (44.8499, -12.8337) knots 0 0 0 1 2 2 2
  line L189 (44.8499, -12.8337) -> (44.8499, -11.3389)
  line L190 (42.9088, -8.991) -> (42.939, -9.3629)
  spline S193 degree 2 poles (42.939, -9.3629) (42.7182, -9.4141) (42.6159, -9.5047) knots 0 0 0 1 1 1
  spline S194 degree 2 poles (42.6159, -9.5047) (42.4555, -9.6582) (42.4555, -9.8813) knots 0 0 0 1 1 1
  spline S195 degree 2 poles (42.4555, -9.8813) (42.4555, -10.0603) (42.5554, -10.1952) knots 0 0 0 1 1 1
  spline S196 degree 2 poles (42.5554, -10.1952) (42.6833, -10.3719) (43.1808, -10.5764) (43.6387, -10.5811) knots 0 0 0 1 2 2 2
  spline S197 degree 2 poles (43.6387, -10.5811) (43.4318, -10.4462) (43.2319, -10.0534) (43.2319, -9.8395) knots 0 0 0 1 2 2 2
  spline S198 degree 2 poles (43.2319, -9.8395) (43.2319, -9.4652) (43.7829, -8.9375) (44.2199, -8.9375) knots 0 0 0 1 2 2 2
  spline S199 degree 2 poles (44.2199, -8.9375) (44.5058, -8.9375) (44.9987, -9.1863) (45.2614, -9.6187) (45.2614, -9.893) knots 0 0 0 1 2 3 3 3
  spline S200 degree 2 poles (45.2614, -9.893) (45.2614, -10.3626) (44.5733, -10.953) (43.7829, -10.953) knots 0 0 0 1 2 2 2
  spline S201 degree 2 poles (43.7829, -10.953) (42.8995, -10.953) (42.4973, -10.6252) knots 0 0 0 1 1 1
  spline S202 degree 2 poles (42.4973, -10.6252) (42.1486, -10.3416) (42.1486, -9.8581) knots 0 0 0 1 1 1
  spline S203 degree 2 poles (42.1486, -9.8581) (42.1486, -9.4978) (42.5531, -9.0375) (42.9088, -8.991) knots 0 0 0 1 2 2 2
  spline S204 degree 2 poles (44.2222, -10.523) (44.4152, -10.523) (44.7685, -10.3579) (44.9545, -10.065) (44.9545, -9.9023) knots 0 0 0 1 2 3 3 3
  spline S205 degree 2 poles (44.9545, -9.9023) (44.9545, -9.6628) (44.5709, -9.3234) (44.2432, -9.3234) knots 0 0 0 1 2 2 2
  spline S206 degree 2 poles (44.2432, -9.3234) (43.927, -9.3234) (43.562, -9.6582) (43.562, -9.9162) knots 0 0 0 1 2 2 2
  spline S207 degree 2 poles (43.562, -9.9162) (43.562, -10.1696) (43.927, -10.523) (44.2222, -10.523) knots 0 0 0 1 2 2 2
  line L191 (44.8499, -4.2347) -> (45.2102, -4.2347)
  line L192 (45.2102, -4.2347) -> (45.2102, -6.2502)
  spline S208 degree 2 poles (45.2102, -6.2502) (45.0754, -6.2548) (44.9499, -6.206) knots 0 0 0 1 1 1
  spline S209 degree 2 poles (44.9499, -6.206) (44.743, -6.1293) (44.3454, -5.7899) (44.0827, -5.4691) knots 0 0 0 1 2 2 2
  spline S210 degree 2 poles (44.0827, -5.4691) (43.6736, -4.9739) (43.1994, -4.6252) (42.9855, -4.6252) knots 0 0 0 1 2 2 2
  spline S211 degree 2 poles (42.9855, -4.6252) (42.7623, -4.6252) (42.4578, -4.9437) (42.4578, -5.1994) knots 0 0 0 1 2 2 2
  spline S212 degree 2 poles (42.4578, -5.1994) (42.4578, -5.4691) (42.7832, -5.7922) (43.0692, -5.7945) knots 0 0 0 1 2 2 2
  line L193 (43.0692, -5.7945) -> (43.0297, -6.1804)
  spline S213 degree 2 poles (43.0297, -6.1804) (42.5996, -6.1409) (42.1486, -5.6248) (42.1486, -5.1901) knots 0 0 0 1 2 2 2
  spline S214 degree 2 poles (42.1486, -5.1901) (42.1486, -4.7507) (42.6345, -4.2393) (42.9948, -4.2393) knots 0 0 0 1 2 2 2
  spline S215 degree 2 poles (42.9948, -4.2393) (43.1784, -4.2393) (43.5318, -4.3881) (43.9223, -4.7368) (44.2641, -5.139) knots 0 0 0 1 2 3 3 3
  spline S216 degree 2 poles (44.2641, -5.139) (44.5454, -5.476) (44.7476, -5.6667) (44.8499, -5.7294) knots 0 0 0 1 2 2 2
  line L194 (44.8499, -5.7294) -> (44.8499, -4.2347)
  line L195 (42.5601, -3.8069) -> (42.1997, -3.8069)
  line L196 (42.1997, -3.8069) -> (42.1997, -1.8333)
  line L197 (42.1997, -1.8333) -> (42.4903, -1.8333)
  spline S217 degree 2 poles (42.4903, -1.8333) (42.8018, -2.1238) (43.8294, -2.6957) (44.371, -2.8515) knots 0 0 0 1 2 2 2
  spline S218 degree 2 poles (44.371, -2.8515) (44.7546, -2.9654) (45.2102, -2.9956) knots 0 0 0 1 1 1
  line L198 (45.2102, -2.9956) -> (45.2102, -3.3815)
  spline S219 degree 2 poles (45.2102, -3.3815) (44.8499, -3.3745) (43.8317, -3.1049) (42.8855, -2.6004) (42.5601, -2.3145) knots 0 0 0 1 2 3 3 3
  line L199 (42.5601, -2.3145) -> (42.5601, -3.8069)
  line L200 (44.8499, 0.5031) -> (45.2102, 0.5031)
  line L201 (45.2102, 0.5031) -> (45.2102, -1.5124)
  spline S220 degree 2 poles (45.2102, -1.5124) (45.0754, -1.5171) (44.9499, -1.4683) knots 0 0 0 1 1 1
  spline S221 degree 2 poles (44.9499, -1.4683) (44.743, -1.3916) (44.3454, -1.0522) (44.0827, -0.7313) knots 0 0 0 1 2 2 2
  spline S222 degree 2 poles (44.0827, -0.7313) (43.6736, -0.2362) (43.1994, 0.1125) (42.9855, 0.1125) knots 0 0 0 1 2 2 2
  spline S223 degree 2 poles (42.9855, 0.1125) (42.7623, 0.1125) (42.4578, -0.206) (42.4578, -0.4617) knots 0 0 0 1 2 2 2
  spline S224 degree 2 poles (42.4578, -0.4617) (42.4578, -0.7313) (42.7832, -1.0545) (43.0692, -1.0568) knots 0 0 0 1 2 2 2
  line L202 (43.0692, -1.0568) -> (43.0297, -1.4427)
  spline S225 degree 2 poles (43.0297, -1.4427) (42.5996, -1.4032) (42.1486, -0.8871) (42.1486, -0.4524) knots 0 0 0 1 2 2 2
  spline S226 degree 2 poles (42.1486, -0.4524) (42.1486, -0.013) (42.6345, 0.4984) (42.9948, 0.4984) knots 0 0 0 1 2 2 2
  spline S227 degree 2 poles (42.9948, 0.4984) (43.1784, 0.4984) (43.5318, 0.3496) (43.9223, 0.0009) (44.2641, -0.4012) knots 0 0 0 1 2 3 3 3
  spline S228 degree 2 poles (44.2641, -0.4012) (44.5454, -0.7383) (44.7476, -0.9289) (44.8499, -0.9917) knots 0 0 0 1 2 2 2
  line L203 (44.8499, -0.9917) -> (44.8499, 0.5031)
  line L204 (42.5601, 0.9308) -> (42.1997, 0.9308)
  line L205 (42.1997, 0.9308) -> (42.1997, 2.9045)
  line L206 (42.1997, 2.9045) -> (42.4903, 2.9045)
  spline S229 degree 2 poles (42.4903, 2.9045) (42.8018, 2.6139) (43.8294, 2.042) (44.371, 1.8863) knots 0 0 0 1 2 2 2
  spline S230 degree 2 poles (44.371, 1.8863) (44.7546, 1.7724) (45.2102, 1.7421) knots 0 0 0 1 1 1
  line L207 (45.2102, 1.7421) -> (45.2102, 1.3562)
  spline S231 degree 2 poles (45.2102, 1.3562) (44.8499, 1.3632) (43.8317, 1.6329) (42.8855, 2.1373) (42.5601, 2.4233) knots 0 0 0 1 2 3 3 3
  line L208 (42.5601, 2.4233) -> (42.5601, 0.9308)
  line L209 (44.8499, 5.2408) -> (45.2102, 5.2408)
  line L210 (45.2102, 5.2408) -> (45.2102, 3.2253)
  spline S232 degree 2 poles (45.2102, 3.2253) (45.0754, 3.2206) (44.9499, 3.2695) knots 0 0 0 1 1 1
  spline S233 degree 2 poles (44.9499, 3.2695) (44.743, 3.3462) (44.3454, 3.6856) (44.0827, 4.0064) knots 0 0 0 1 2 2 2
  spline S234 degree 2 poles (44.0827, 4.0064) (43.6736, 4.5015) (43.1994, 4.8502) (42.9855, 4.8502) knots 0 0 0 1 2 2 2
  spline S235 degree 2 poles (42.9855, 4.8502) (42.7623, 4.8502) (42.4578, 4.5318) (42.4578, 4.276) knots 0 0 0 1 2 2 2
  spline S236 degree 2 poles (42.4578, 4.276) (42.4578, 4.0064) (42.7832, 3.6832) (43.0692, 3.6809) knots 0 0 0 1 2 2 2
  line L211 (43.0692, 3.6809) -> (43.0297, 3.295)
  spline S237 degree 2 poles (43.0297, 3.295) (42.5996, 3.3345) (42.1486, 3.8506) (42.1486, 4.2853) knots 0 0 0 1 2 2 2
  spline S238 degree 2 poles (42.1486, 4.2853) (42.1486, 4.7247) (42.6345, 5.2361) (42.9948, 5.2361) knots 0 0 0 1 2 2 2
  spline S239 degree 2 poles (42.9948, 5.2361) (43.1784, 5.2361) (43.5318, 5.0874) (43.9223, 4.7387) (44.2641, 4.3365) knots 0 0 0 1 2 3 3 3
  spline S240 degree 2 poles (44.2641, 4.3365) (44.5454, 3.9994) (44.7476, 3.8088) (44.8499, 3.746) knots 0 0 0 1 2 2 2
  line L212 (44.8499, 3.746) -> (44.8499, 5.2408)
  line L213 (44.5035, 5.6988) -> (44.471, 6.0591)
  spline S241 degree 2 poles (44.471, 6.0591) (44.7244, 6.1056) (44.9545, 6.3636) (44.9545, 6.5635) knots 0 0 0 1 2 2 2
  spline S242 degree 2 poles (44.9545, 6.5635) (44.9545, 6.7356) (44.7964, 6.9983) (44.5314, 7.1633) (44.0827, 7.2749) (43.848, 7.2749) knots 0 0 0 1 2 3 4 4 4
  spline S243 degree 2 poles (43.848, 7.2749) (43.8247, 7.2749) (43.7736, 7.2726) knots 0 0 0 1 1 1
  spline S244 degree 2 poles (43.7736, 7.2726) (43.9526, 7.161) (44.1757, 6.7728) (44.1757, 6.5449) knots 0 0 0 1 2 2 2
  spline S245 degree 2 poles (44.1757, 6.5449) (44.1757, 6.166) (43.6271, 5.643) (43.1784, 5.643) knots 0 0 0 1 2 2 2
  spline S246 degree 2 poles (43.1784, 5.643) (42.7135, 5.643) (42.1486, 6.1893) (42.1486, 6.6007) knots 0 0 0 1 2 2 2
  spline S247 degree 2 poles (42.1486, 6.6007) (42.1486, 6.8983) (42.4694, 7.3911) (43.0622, 7.6469) (43.6225, 7.6469) knots 0 0 0 1 2 3 3 3
  spline S248 degree 2 poles (43.6225, 7.6469) (44.2083, 7.6469) (44.8987, 7.3935) (45.2614, 6.8913) (45.2614, 6.5542) knots 0 0 0 1 2 3 3 3
  spline S249 degree 2 poles (45.2614, 6.5542) (45.2614, 6.1986) (44.8638, 5.7453) (44.5035, 5.6988) knots 0 0 0 1 2 2 2
  spline S250 degree 2 poles (43.1598, 7.2307) (42.8367, 7.2307) (42.4578, 6.889) (42.4578, 6.6472) knots 0 0 0 1 2 2 2
  spline S251 degree 2 poles (42.4578, 6.6472) (42.4578, 6.3962) (42.8646, 6.0289) (43.1901, 6.0289) knots 0 0 0 1 2 2 2
  spline S252 degree 2 poles (43.1901, 6.0289) (43.4807, 6.0289) (43.8456, 6.3776) (43.8456, 6.6379) knots 0 0 0 1 2 2 2
  spline S253 degree 2 poles (43.8456, 6.6379) (43.8456, 6.896) (43.4807, 7.2307) (43.1598, 7.2307) knots 0 0 0 1 2 2 2
  line L214 (44.8499, 11.1618) -> (45.2102, 11.1618)
  line L215 (45.2102, 11.1618) -> (45.2102, 9.1463)
  spline S254 degree 2 poles (45.2102, 9.1463) (45.0754, 9.1416) (44.9499, 9.1905) knots 0 0 0 1 1 1
  spline S255 degree 2 poles (44.9499, 9.1905) (44.743, 9.2672) (44.3454, 9.6066) (44.0827, 9.9274) knots 0 0 0 1 2 2 2
  spline S256 degree 2 poles (44.0827, 9.9274) (43.6736, 10.4225) (43.1994, 10.7712) (42.9855, 10.7712) knots 0 0 0 1 2 2 2
  spline S257 degree 2 poles (42.9855, 10.7712) (42.7623, 10.7712) (42.4578, 10.4528) (42.4578, 10.197) knots 0 0 0 1 2 2 2
  spline S258 degree 2 poles (42.4578, 10.197) (42.4578, 9.9274) (42.7832, 9.6042) (43.0692, 9.6019) knots 0 0 0 1 2 2 2
  line L216 (43.0692, 9.6019) -> (43.0297, 9.216)
  spline S259 degree 2 poles (43.0297, 9.216) (42.5996, 9.2555) (42.1486, 9.7716) (42.1486, 10.2063) knots 0 0 0 1 2 2 2
  spline S260 degree 2 poles (42.1486, 10.2063) (42.1486, 10.6457) (42.6345, 11.1571) (42.9948, 11.1571) knots 0 0 0 1 2 2 2
  spline S261 degree 2 poles (42.9948, 11.1571) (43.1784, 11.1571) (43.5318, 11.0084) (43.9223, 10.6597) (44.2641, 10.2575) knots 0 0 0 1 2 3 3 3
  spline S262 degree 2 poles (44.2641, 10.2575) (44.5454, 9.9204) (44.7476, 9.7298) (44.8499, 9.667) knots 0 0 0 1 2 2 2
  line L217 (44.8499, 9.667) -> (44.8499, 11.1618)
  line L218 (42.5601, 11.5895) -> (42.1997, 11.5895)
  line L219 (42.1997, 11.5895) -> (42.1997, 13.5632)
  line L220 (42.1997, 13.5632) -> (42.4903, 13.5632)
  spline S263 degree 2 poles (42.4903, 13.5632) (42.8018, 13.2726) (43.8294, 12.7007) (44.371, 12.545) knots 0 0 0 1 2 2 2
  spline S264 degree 2 poles (44.371, 12.545) (44.7546, 12.4311) (45.2102, 12.4009) knots 0 0 0 1 1 1
  line L221 (45.2102, 12.4009) -> (45.2102, 12.015)
  spline S265 degree 2 poles (45.2102, 12.015) (44.8499, 12.0219) (43.8317, 12.2916) (42.8855, 12.7961) (42.5601, 13.082) knots 0 0 0 1 2 3 3 3
  line L222 (42.5601, 13.082) -> (42.5601, 11.5895)
  line L223 (44.8499, 15.8995) -> (45.2102, 15.8995)
  line L224 (45.2102, 15.8995) -> (45.2102, 13.884)
  spline S266 degree 2 poles (45.2102, 13.884) (45.0754, 13.8794) (44.9499, 13.9282) knots 0 0 0 1 1 1
  spline S267 degree 2 poles (44.9499, 13.9282) (44.743, 14.0049) (44.3454, 14.3443) (44.0827, 14.6651) knots 0 0 0 1 2 2 2
  spline S268 degree 2 poles (44.0827, 14.6651) (43.6736, 15.1603) (43.1994, 15.509) (42.9855, 15.509) knots 0 0 0 1 2 2 2
  spline S269 degree 2 poles (42.9855, 15.509) (42.7623, 15.509) (42.4578, 15.1905) (42.4578, 14.9348) knots 0 0 0 1 2 2 2
  spline S270 degree 2 poles (42.4578, 14.9348) (42.4578, 14.6651) (42.7832, 14.342) (43.0692, 14.3397) knots 0 0 0 1 2 2 2
  line L225 (43.0692, 14.3397) -> (43.0297, 13.9538)
  spline S271 degree 2 poles (43.0297, 13.9538) (42.5996, 13.9933) (42.1486, 14.5094) (42.1486, 14.9441) knots 0 0 0 1 2 2 2
  spline S272 degree 2 poles (42.1486, 14.9441) (42.1486, 15.3834) (42.6345, 15.8949) (42.9948, 15.8949) knots 0 0 0 1 2 2 2
  spline S273 degree 2 poles (42.9948, 15.8949) (43.1784, 15.8949) (43.5318, 15.7461) (43.9223, 15.3974) (44.2641, 14.9952) knots 0 0 0 1 2 3 3 3
  spline S274 degree 2 poles (44.2641, 14.9952) (44.5454, 14.6581) (44.7476, 14.4675) (44.8499, 14.4047) knots 0 0 0 1 2 2 2
  line L226 (44.8499, 14.4047) -> (44.8499, 15.8995)
  line L227 (42.9088, 18.2475) -> (42.939, 17.8755)
  spline S275 degree 2 poles (42.939, 17.8755) (42.7182, 17.8244) (42.6159, 17.7337) knots 0 0 0 1 1 1
  spline S276 degree 2 poles (42.6159, 17.7337) (42.4555, 17.5803) (42.4555, 17.3571) knots 0 0 0 1 1 1
  spline S277 degree 2 poles (42.4555, 17.3571) (42.4555, 17.1781) (42.5554, 17.0433) knots 0 0 0 1 1 1
  spline S278 degree 2 poles (42.5554, 17.0433) (42.6833, 16.8666) (43.1808, 16.662) (43.6387, 16.6574) knots 0 0 0 1 2 2 2
  spline S279 degree 2 poles (43.6387, 16.6574) (43.4318, 16.7922) (43.2319, 17.1851) (43.2319, 17.399) knots 0 0 0 1 2 2 2
  spline S280 degree 2 poles (43.2319, 17.399) (43.2319, 17.7732) (43.7829, 18.3009) (44.2199, 18.3009) knots 0 0 0 1 2 2 2
  spline S281 degree 2 poles (44.2199, 18.3009) (44.5058, 18.3009) (44.9987, 18.0522) (45.2614, 17.6198) (45.2614, 17.3455) knots 0 0 0 1 2 3 3 3
  spline S282 degree 2 poles (45.2614, 17.3455) (45.2614, 16.8759) (44.5733, 16.2854) (43.7829, 16.2854) knots 0 0 0 1 2 2 2
  spline S283 degree 2 poles (43.7829, 16.2854) (42.8995, 16.2854) (42.4973, 16.6132) knots 0 0 0 1 1 1
  spline S284 degree 2 poles (42.4973, 16.6132) (42.1486, 16.8968) (42.1486, 17.3804) knots 0 0 0 1 1 1
  spline S285 degree 2 poles (42.1486, 17.3804) (42.1486, 17.7407) (42.5531, 18.201) (42.9088, 18.2475) knots 0 0 0 1 2 2 2